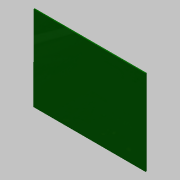
# Autodesk Inventor part: Brain_demo_PCB
Saved by Autodesk Inventor 2019.3 (Build 233278000, 278)
## iProperties
Created: 2019-04-15
Part Number: Brain_demo_PCB
Material: Generic
Document SubType Name: Modeling
Designer: Varga Daniel
Density: 1 g/cm^3
Appearance: PCB color
Author: Varga Daniel
Autodesk Inventor part; units mm, degrees
ref_plane "YZ Plane" through (0, 0, 0) normal (1, 0, 0) x (0, 1, 0)
ref_plane "XZ Plane" through (0, 0, 0) normal (0, 1, 0) x (-1, 0, 0)
ref_plane "XY Plane" through (0, 0, 0) normal (0, 0, 1) x (1, 0, 0)
sketch "Sketch1" plane through (0, 0, 0) normal (0, 0, 1) x (1, 0, 0)
  line L0 (0, 0) -> (-102.2, 0) construction
  line L1 (4.8, 0.2) -> (-3.2, 0.2) construction
  line L2 (-102.6844, -6.0028) -> (-100.5, -6.0028) construction
  line L3 (-100.5, -6.0028) -> (-100.5, -3.2528) construction
  arc A0 (-97.5, -3.2528) -> (-100.5, -3.2528) centre (-99, -3.2528) ccw construction
  line L4 (-97.5, -3.2528) -> (-97.5, -6.0028) construction
  line L5 (-97.5, -6.0028) -> (-96.2, -6.0028) construction
  line L6 (-96.2, -6.0028) -> (-96.2, -0.5028) construction
  line L7 (-96.2, -0.5028) -> (-5.5, -0.5028) construction
  line L8 (-5.5, -0.5028) -> (-5.5, -6.0028) construction
  line L9 (-5.5, -6.0028) -> (-4.25, -6.0028) construction
  line L10 (-4.25, -6.0028) -> (-4.25, -3.2528) construction
  arc A1 (-1.25, -3.2528) -> (-4.25, -3.2528) centre (-2.75, -3.2528) ccw construction
  line L11 (-1.25, -3.2528) -> (-1.25, -6.0028) construction
  line L12 (-1.25, -6.0028) -> (0, -6.0028) construction
  line L13 (0, 0) -> (0, -6.0028) construction
  line L14 (-102.2, 0) -> (0, 0) construction
  arc A2 (-102.2, 0) -> (-102.6844, -0.1251) centre (-102.2, -1) ccw construction
  line L15 (-102.6844, -0.1251) -> (-102.6844, -6.0028) construction
  line L16 (-100.5, -72.0028) -> (-102.6844, -72.0028) construction
  line L17 (-102.6844, -72.0028) -> (-102.6844, -77.8749) construction
  arc A3 (-102.6844, -77.8749) -> (-102.2, -78) centre (-102.2, -77) ccw construction
  line L18 (0, -78) -> (-102.2, -78) construction
  line L19 (0, -72.0028) -> (0, -78) construction
  line L20 (0, -72.0028) -> (-1.25, -72.0028) construction
  line L21 (-1.25, -72.0028) -> (-1.25, -74.7528) construction
  arc A4 (-4.25, -74.7528) -> (-1.25, -74.7528) centre (-2.75, -74.7528) ccw construction
  line L22 (-4.25, -74.7528) -> (-4.25, -72.0028) construction
  line L23 (-4.25, -72.0028) -> (-5.5, -72.0028) construction
  line L24 (-5.5, -72.0028) -> (-5.5, -77.5028) construction
  line L25 (-5.5, -77.5028) -> (-96.2, -77.5028) construction
  line L26 (-96.2, -77.5028) -> (-96.2, -72.0028) construction
  line L27 (-96.2, -72.0028) -> (-97.5, -72.0028) construction
  line L28 (-97.5, -72.0028) -> (-97.5, -74.7528) construction
  arc A5 (-100.5, -74.7528) -> (-97.5, -74.7528) centre (-99, -74.7528) ccw construction
  line L29 (-100.5, -74.7528) -> (-100.5, -72.0028) construction
  line L30 (0, -78) -> (-102.6844, -77.8749)
  line L31 (-102.6844, -77.8749) -> (-102.4501, -0.0318)
  line L32 (-102.4501, -0.0318) -> (0, 0)
  line L33 (0, 0) -> (0, -78)
  constraints: 8 end point, 1 point on circle
extrude "Extrusion1" add sketch "Sketch1" along normal blind 1
body "Solid1"
